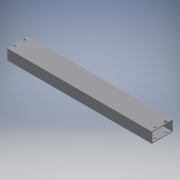
# Autodesk Inventor part: Tube
Saved by Autodesk Inventor 2016 (Build 200138000, 138)
## iProperties
Created: 2017-01-08
Part Number: Tube
Material: Generic
Document SubType Name: Modeling
Designer: Dhruv
Density: 1 g/cm^3
Appearance: Default
Author: Dhruv
Autodesk Inventor part; units mm, degrees
ref_plane "YZ Plane" through (0, 0, 0) normal (1, 0, 0) x (0, 1, 0)
ref_plane "XZ Plane" through (0, 0, 0) normal (0, 1, 0) x (-1, 0, 0)
ref_plane "XY Plane" through (0, 0, 0) normal (0, 0, 1) x (1, 0, 0)
sketch "Sketch1" plane through (0, 0, 0) normal (0, 1, 0) x (-1, 0, 0)
  line L0 (176.1109, -25.4) -> (-176.1109, -25.4)
  line L1 (-176.1109, -25.4) -> (-176.1109, 25.4)
  line L2 (-176.1109, 25.4) -> (176.1109, 25.4)
  line L3 (176.1109, 25.4) -> (176.1109, -25.4)
  line L4 (176.1109, -25.4) -> (-176.1109, 25.4) construction
  line L5 (-176.1109, -25.4) -> (176.1109, 25.4) construction
  point P0 (0, 0)
  dimension "d0" = 352.2218
  dimension "d1" = 50.8
  constraints: 12 end point, 2 midpoint, 2 parallel, 1 horizontal, 1 perpendicular
  measures "d0" distance of L1.end L2.end
  measures "d1" distance of L0.end L1.end
extrude "Extrusion1" add sketch "Sketch1" along normal blind 25.4
sketch "Sketch2" plane through (176.1109, 0, 25.4) normal (1, 0, 0) x (0, 0, -1)
  line L0 (25.4, 0) -> (25.4, 12.7) construction
  line L1 (1.5875, 23.8125) -> (49.2125, 23.8125)
  line L2 (49.2125, 23.8125) -> (49.2125, 1.5875)
  line L3 (49.2125, 1.5875) -> (1.5875, 1.5875)
  line L4 (1.5875, 1.5875) -> (1.5875, 23.8125)
  line L5 (1.5875, 23.8125) -> (49.2125, 1.5875) construction
  line L6 (49.2125, 23.8125) -> (1.5875, 1.5875) construction
  dimension "d4" = 12.7
  dimension "d5" = 47.625
  dimension "d6" = 22.225
  constraints: 14 end point, 2 midpoint, 2 parallel, 1 horizontal, 1 perpendicular, 1 vertical
  measures "d4" distance of L0.start L0.end
  measures "d5" distance of L2.end L3.end
  measures "d6" distance of L1.end L2.end
extrude "Extrusion2" cut sketch "Sketch2" against normal through all
sketch "Sketch3" plane through (0, 25.4, 0) normal (0, 1, 0) x (1, 0, 0)
  line L0 (-180.7718, 12.7) -> (-171.45, 12.7) construction
  line L1 (-171.45, 12.7) -> (-171.45, -12.7) construction
  line L2 (-171.45, -12.7) -> (-180.7718, -12.7) construction
  line L3 (-180.7718, -12.7) -> (-180.7718, 12.7) construction
  line L4 (-176.1109, 23.8125) -> (-176.1109, -23.8125) construction
  line L5 (-180.7718, 12.7) -> (-171.45, -12.7) construction
  line L6 (-171.45, 12.7) -> (-180.7718, -12.7) construction
  circle A0 centre (-171.45, 12.7) radius 3.175
  circle A1 centre (-171.45, -12.7) radius 3.175
  line L7 (0, 0) -> (0, -23.8125) construction
  circle A2 centre (171.45, 12.7) radius 3.175
  circle A3 centre (171.45, -12.7) radius 3.175
  point P0 (-176.1109, 0)
  dimension "d9" = 9.3218
  dimension "d10" = 25.4
  dimension "d11" = 6.35
  dimension "d12" = 6.35
  constraints: 14 end point, 4 centre point, 3 midpoint, 2 coincident, 2 parallel, 2 symmetric about line, 1 horizontal, 1 perpendicular, 1 vertical, 2 other
  measures "d9" distance of L1.end L2.end
  measures "d10" distance of L0.end L1.end
  measures "d11" diameter of A0
  measures "d12" diameter of A1
extrude "Extrusion3" cut sketch "Sketch3" against normal through all
body "Solid1"
